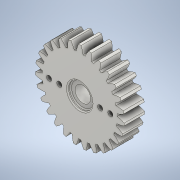
# Autodesk Inventor part: шестерня_1
Saved by Autodesk Inventor 2022 (Build 260153000, 153)
## iProperties
CustomPartVersion: 1
Created: 2022-12-27
Part Number: шестерня_1
Material: Steel
Document SubType Name: Modeling
Designer: Pavel
Categories: <?xml version="1.0" encoding="UTF-16"?> <MemberInstance><Categories><FamilyTemplate><FamilyTemplateParameter ValueType="xs:double" Id="1" ObjectReferenceKey="da_z" ObjectType="kUserParameterObject"/><FamilyTemplateParameter ValueType="xs:double" Id="2" ObjectReferenceKey="da_b" ObjectType="kUserParameterObject"/><FamilyTemplateParameter ValueType="xs:double" Id="3" ObjectReferenceKey="da_beta" ObjectType="kUserParameterObject"/><FamilyTemplateParameter ValueType="xs:double" Id="4" ObjectReferenceKey="da_da" ObjectType="kUserParameterObject"/><FamilyTemplateParameter ValueType="xs:double" Id="5" ObjectReferenceKey="da_aw" ObjectType="kUserParameterObject"/><FamilyTemplateParameter ValueType="xs:string" Id="6" ObjectReferenceKey="EAIAABAAAACIAQAAAAAAAIAAAAAAAAAA" ObjectType="83910656" SubObjectId="SurfaceGeometry"/></FamilyTemplate><ParamToTemplateMap><ParamToTemplate CategoryParameter="//CategoryParameter[@InternalName='046C89C9-8512-4d59-83FE-43B91F4F132A']" TemplateParameter="1"/><ParamToTemplate CategoryParameter="//CategoryParameter[@InternalName='2552DF32-E462-4b46-AEBF-C6C7768E72AC']" TemplateParameter="2"/><ParamToTemplate CategoryParameter="//CategoryParameter[@InternalName='C9EE641D-15FC-4fae-A226-E94C4372FDD7']" TemplateParameter="3"/><ParamToTemplate><ParamToTemplate CategoryParameter="//CategoryParameter[@InternalName='00B6519A-459B-49c7-AD84-2E56D39A5744']" ConstantValue="0.000000"/></ParamToTemplate><ParamToTemplate><ParamToTemplate CategoryParameter="//CategoryParameter[@InternalName='04B31F0E-C7A6-4894-AA32-9629BEFACF47']" ConstantValue="1.000000"/></ParamToTemplate><ParamToTemplate><ParamToTemplate CategoryParameter="//CategoryParameter[@InternalName='43CBEC2E-7847-49e7-A936-2F7889FCB2D9']" ConstantValue="0.250000"/></ParamToTemplate><ParamToTemplate><ParamToTemplate CategoryParameter="//CategoryParameter[@InternalName='B1EFC894-105D-4ebd-86BF-FA20ED196853']" ConstantValue="0.350000"/></ParamToTemplate><ParamToTemplate><ParamToTemplate CategoryParameter="//CategoryParameter[@InternalName='51175063-3D10-4879-93E8-6246FE8B403D']" ConstantValue="2060000000.000000"/></ParamToTemplate><ParamToTemplate><ParamToTemplate CategoryParameter="//CategoryParameter[@InternalName='A3A52E27-4454-46a9-B0BD-C932399B70AF']" ConstantValue="0.300000"/></ParamToTemplate><ParamToTemplate><ParamToTemplate CategoryParameter="//CategoryParameter[@InternalName='91B76062-C214-41d9-B1B9-14D2AB99603D']" ConstantValue="0.150000"/></ParamToTemplate><ParamToTemplate><ParamToTemplate CategoryParameter="//CategoryParameter[@InternalName='374E806E-8B8A-4dda-A9AA-1039D6500AD2']" ConstantValue="6.666667"/></ParamToTemplate><ParamToTemplate><ParamToTemplate CategoryParameter="//CategoryParameter[@InternalName='2D373A89-B862-43d6-8D0B-0CBF12AB9F6C']" ConstantValue="0.349066"/></ParamToTemplate><ParamToTemplate CategoryParameter="//CategoryParameter[@InternalName='37777632-D6A2-4fac-9D53-DB8ACD95C989']" TemplateParameter="4"/><ParamToTemplate CategoryParameter="//CategoryParameter[@InternalName='FD1017F1-B727-4f7e-9707-0F86F1FF9423']" TemplateParameter="5"/><ParamToTemplate><ParamToTemplate CategoryParameter="//CategoryParameter[@InternalName='9E1B4470-B2D3-4ff1-B813-535BB4CDF51A']" ConstantValue="3520000.000000"/></ParamToTemplate><ParamToTemplate><ParamToTemplate CategoryParameter="//CategoryParameter[@InternalName='F8452263-BFF6-458c-9FB1-07C4B99E95CD']" ConstantValue="11400000.000000"/></ParamToTemplate><ParamToTemplate><ParamToTemplate CategoryParameter="//CategoryParameter[@InternalName='3E3BB259-FD49-497f-8171-6EBC954A3479']" ConstantValue="2.000000"/></ParamToTemplate><ParamToTemplate CategoryParameter="//CategoryParameter[@InternalName='27C3BAF2-7550-4e4b-AE2C-0DB134B7D9B7']" TemplateParameter="6"/></ParamToTemplateMap><Category DisplayName="Gear" InternalName="DC85795E-93AB-48d5-8EEE-5A27447B64BD" Mnemonic="Gear"><CategoryParameter DisplayName="z" InternalName="046C89C9-8512-4d59-83FE-43B91F4F132A" Mnemonic="z"/><CategoryParameter DisplayName="b" InternalName="2552DF32-E462-4b46-AEBF-C6C7768E72AC" Mnemonic="b"/><CategoryParameter DisplayName="||b|" InternalName="C9EE641D-15FC-4fae-A226-E94C4372FDD7" Mnemonic="beta"/><CategoryParameter DisplayName="x" InternalName="00B6519A-459B-49c7-AD84-2E56D39A5744" Mnemonic="x"/><CategoryParameter DisplayName="a*" InternalName="04B31F0E-C7A6-4894-AA32-9629BEFACF47" Mnemonic="a"/><CategoryParameter DisplayName="c*" InternalName="43CBEC2E-7847-49e7-A936-2F7889FCB2D9" Mnemonic="c"/><CategoryParameter DisplayName="r|.f|*" InternalName="B1EFC894-105D-4ebd-86BF-FA20ED196853" Mnemonic="rf"/><CategoryParameter DisplayName="E" InternalName="51175063-3D10-4879-93E8-6246FE8B403D" Mnemonic="E"/><CategoryParameter DisplayName="||m|" InternalName="A3A52E27-4454-46a9-B0BD-C932399B70AF" Mnemonic="mi"/><Category DisplayName="SpurGear" InternalName="26C5A22E-A91E-4dfd-A3B3-23CCAFAE1764" Mnemonic="SpurGear"><CategoryParameter DisplayName="m" InternalName="91B76062-C214-41d9-B1B9-14D2AB99603D" Mnemonic="m"/><CategoryParameter DisplayName="P" InternalName="374E806E-8B8A-4dda-A9AA-1039D6500AD2" Mnemonic="PP"/><CategoryParameter DisplayName="||a|" InternalName="2D373A89-B862-43d6-8D0B-0CBF12AB9F6C" Mnemonic="alpha"/><CategoryParameter DisplayName="d|.a|" InternalName="37777632-D6A2-4fac-9D53-DB8ACD95C989" Mnemonic="da"/><CategoryParameter DisplayName="a|.w|" InternalName="FD1017F1-B727-4f7e-9707-0F86F1FF9423" Mnemonic="aw"/><CategoryParameter DisplayName="||s||.Flim|" InternalName="9E1B4470-B2D3-4ff1-B813-535BB4CDF51A" Mnemonic="sFlim"/><CategoryParameter DisplayName="||s||.Hlim|" InternalName="F8452263-BFF6-458c-9FB1-07C4B99E95CD" Mnemonic="sHlim"/><CategoryParameter DisplayName="тип" InternalName="3E3BB259-FD49-497f-8171-6EBC954A3479" Mnemonic="type"/><CategoryParameter DisplayName="PitchDiameter" InternalName="27C3BAF2-7550-4e4b-AE2C-0DB134B7D9B7" Mnemonic="IDS_PITCHDIAM"/></Category></Category></Categories></MemberInstance>
Density: 1 g/cm^3
Appearance: Steel
Author: Pavel
Autodesk Inventor part; units mm, degrees
ref_plane "YZ Plane" through (0, 0, 0) normal (1, 0, 0) x (0, 1, 0)
ref_plane "XZ Plane" through (0, 0, 0) normal (0, 1, 0) x (-1, 0, 0)
ref_plane "XY Plane" through (0, 0, 0) normal (0, 0, 1) x (1, 0, 0)
sketch "Sketch1" plane through (0, 0, 0) normal (0, 0, 1) x (1, 0, 0)
  circle A0 centre (0, 0) radius 21.7404
  dimension "d0" = 43.4808
  constraints: 1 centre point
  measures "d0" diameter of A0
extrude "Extrusion1" add sketch "Sketch1" along normal blind 6
ref_plane "Work Plane2" through (0, 0, 3) normal (0, 0, 1) x (1, 0, 0)
sketch "Sketch2" plane through (0, 0, 0) normal (0, 0, -1) x (-1, 0, 0)
  circle A0 centre (0, 0) radius 21.7404 projected
  circle A1 centre (0, 0) radius 20.25
  dimension "d3" = 40.5
  constraints: 1 centre point, 1 coincident
  measures "d3" diameter of A1
surface extrude "Средний диаметр" sketch "Sketch2" against normal through all shown no curves A1
ref_plane "Work Plane8" through (0, 0, 0) normal (0.9932384, 0.1160929, 0) x (0, 0, 1)
ref_plane "Work Plane9" through (0, 0, 0) normal (1, 0, 0) x (0, 1, 0)
spur gear teeth "Цилиндрическое зубчатое зацепление" teeth 27 pitch diameter 40.5 tip diameter 43.4808 root diameter 36.75 face width 6 start plane through (0, 0, 0) normal (0, 0, -1) x (-1, 0, 0)
sketch "Эскиз6" plane through (0, 0, 6) normal (0, 0, 1) x (1, 0, 0)
  arc A0 (-5.6268, 20.9996) -> (-5.7798, 17.4423) centre (8.4688, 18.6117) ccw projected
  arc A1 (-5.7798, 17.4423) -> (-6.7842, 17.0768) centre (0, 0) ccw projected
  arc A2 (-6.7842, 17.0768) -> (-9.1879, 19.7035) centre (-18.4509, 8.8138) ccw projected
  arc A3 (-9.1879, 19.7035) -> (-10.318, 19.1359) centre (0, 0) ccw projected
  arc A4 (-10.318, 19.1359) -> (-9.6464, 15.6393) centre (3.9483, 20.0631) ccw projected
  arc A5 (-9.6464, 15.6393) -> (-10.5395, 15.0519) centre (0, 0) ccw projected
  arc A6 (-10.5395, 15.0519) -> (-13.4842, 17.0535) centre (-19.9861, 4.3212) ccw projected
  arc A7 (-13.4842, 17.0535) -> (-14.4529, 16.2406) centre (0, 0) ccw projected
  arc A8 (-14.4529, 16.2406) -> (-12.9931, 12.9931) centre (-0.785, 20.4328) ccw projected
  arc A9 (-12.9931, 12.9931) -> (-13.7266, 12.2156) centre (0, 0) ccw projected
  arc A10 (-13.7266, 12.2156) -> (-17.0535, 13.4842) centre (-20.4439, -0.4044) ccw projected
  arc A11 (-17.0535, 13.4842) -> (-17.8087, 12.4698) centre (0, 0) ccw projected
  arc A12 (-17.8087, 12.4698) -> (-15.6393, 9.6464) centre (-5.4759, 19.7011) ccw projected
  arc A13 (-15.6393, 9.6464) -> (-16.1737, 8.7208) centre (0, 0) ccw projected
  arc A14 (-16.1737, 8.7208) -> (-19.7035, 9.1879) centre (-19.7996, -5.1082) ccw projected
  arc A15 (-19.7035, 9.1879) -> (-20.2044, 8.0267) centre (0, 0) ccw projected
  arc A16 (-20.2044, 8.0267) -> (-17.4423, 5.7798) centre (-9.8717, 17.9072) ccw projected
  arc A17 (-17.4423, 5.7798) -> (-17.7489, 4.7558) centre (0, 0) ccw projected
  arc A18 (-17.7489, 4.7558) -> (-21.2913, 4.3963) centre (-18.0878, -9.5366) ccw projected
  arc A19 (-21.2913, 4.3963) -> (-21.5109, 3.1509) centre (0, 0) ccw projected
  arc A20 (-21.5109, 3.1509) -> (-18.3051, 1.6015) centre (-13.7353, 15.1479) ccw projected
  arc A21 (-18.3051, 1.6015) -> (-18.3672, 0.5344) centre (0, 0) ccw projected
  arc A22 (-18.3672, 0.5344) -> (-21.7312, -0.6323) centre (-15.401, -13.4509) ccw projected
  arc A23 (-21.7312, -0.6323) -> (-21.6577, -1.8948) centre (0, 0) ccw projected
  arc A24 (-21.6577, -1.8948) -> (-18.181, -2.6631) centre (-16.8584, 11.572) ccw projected
  arc A25 (-18.181, -2.6631) -> (-17.9954, -3.7157) centre (0, 0) ccw projected
  arc A26 (-17.9954, -3.7157) -> (-20.9996, -5.6268) centre (-11.8838, -16.6401) ccw projected
  arc A27 (-20.9996, -5.6268) -> (-20.6369, -6.8383) centre (0, 0) ccw projected
  arc A28 (-20.6369, -6.8383) -> (-17.0768, -6.7842) centre (-19.0727, 7.3723) ccw projected
  arc A29 (-17.0768, -6.7842) -> (-16.6534, -7.7656) centre (0, 0) ccw projected
  arc A30 (-16.6534, -7.7656) -> (-19.1359, -10.318) centre (-7.7261, -18.9321) ccw projected
  arc A31 (-19.1359, -10.318) -> (-18.5036, -11.4132) centre (0, 0) ccw projected
  arc A32 (-18.5036, -11.4132) -> (-15.0519, -10.5395) centre (-20.2587, 2.7751) ccw projected
  arc A33 (-15.0519, -10.5395) -> (-14.4136, -11.3968) centre (0, 0) ccw projected
  arc A34 (-14.4136, -11.3968) -> (-16.2406, -14.4529) centre (-3.1518, -20.2036) ccw projected
  arc A35 (-16.2406, -14.4529) -> (-15.3728, -15.3728) centre (0, 0) ccw projected
  arc A36 (-15.3728, -15.3728) -> (-12.2156, -13.7266) centre (-20.3526, -1.9717) ccw projected
  arc A37 (-12.2156, -13.7266) -> (-11.3968, -14.4136) centre (0, 0) ccw projected
  arc A38 (-11.3968, -14.4136) -> (-12.4698, -17.8087) centre (1.5925, -20.3858) ccw projected
  arc A39 (-12.4698, -17.8087) -> (-11.4132, -18.5036) centre (0, 0) ccw projected
  arc A40 (-11.4132, -18.5036) -> (-8.7208, -16.1737) centre (-19.3493, -6.6122) ccw projected
  arc A41 (-8.7208, -16.1737) -> (-7.7656, -16.6534) centre (0, 0) ccw projected
  arc A42 (-7.7656, -16.6534) -> (-8.0267, -20.2044) centre (6.2508, -19.4691) ccw projected
  arc A43 (-8.0267, -20.2044) -> (-6.8383, -20.6369) centre (0, 0) ccw projected
  arc A44 (-6.8383, -20.6369) -> (-4.7558, -17.7489) centre (-17.3029, -10.8962) ccw projected
  arc A45 (-4.7558, -17.7489) -> (-3.7157, -17.9954) centre (0, 0) ccw projected
  arc A46 (-3.7157, -17.9954) -> (-3.1509, -21.5109) centre (10.5722, -17.5027) ccw projected
  arc A47 (-3.1509, -21.5109) -> (-1.8948, -21.6577) centre (0, 0) ccw projected
  arc A48 (-1.8948, -21.6577) -> (-0.5344, -18.3672) centre (-14.3236, -14.5928) ccw projected
  arc A49 (-0.5344, -18.3672) -> (0.5344, -18.3672) centre (0, 0) ccw projected
  arc A50 (0.5344, -18.3672) -> (1.8948, -21.6577) centre (14.3236, -14.5928) ccw projected
  arc A51 (1.8948, -21.6577) -> (3.1509, -21.5109) centre (0, 0) ccw projected
  arc A52 (3.1509, -21.5109) -> (3.7157, -17.9954) centre (-10.5722, -17.5027) ccw projected
  arc A53 (3.7157, -17.9954) -> (4.7558, -17.7489) centre (0, 0) ccw projected
  arc A54 (4.7558, -17.7489) -> (6.8383, -20.6369) centre (17.3029, -10.8962) ccw projected
  arc A55 (6.8383, -20.6369) -> (8.0267, -20.2044) centre (0, 0) ccw projected
  arc A56 (8.0267, -20.2044) -> (7.7656, -16.6534) centre (-6.2508, -19.4691) ccw projected
  arc A57 (7.7656, -16.6534) -> (8.7208, -16.1737) centre (0, 0) ccw projected
  arc A58 (8.7208, -16.1737) -> (11.4132, -18.5036) centre (19.3493, -6.6122) ccw projected
  arc A59 (11.4132, -18.5036) -> (12.4698, -17.8087) centre (0, 0) ccw projected
  arc A60 (12.4698, -17.8087) -> (11.3968, -14.4136) centre (-1.5925, -20.3858) ccw projected
  arc A61 (11.3968, -14.4136) -> (12.2156, -13.7266) centre (0, 0) ccw projected
  arc A62 (12.2156, -13.7266) -> (15.3728, -15.3728) centre (20.3526, -1.9717) ccw projected
  arc A63 (15.3728, -15.3728) -> (16.2406, -14.4529) centre (0, 0) ccw projected
  arc A64 (16.2406, -14.4529) -> (14.4136, -11.3968) centre (3.1518, -20.2036) ccw projected
  arc A65 (14.4136, -11.3968) -> (15.0519, -10.5395) centre (0, 0) ccw projected
  arc A66 (15.0519, -10.5395) -> (18.5036, -11.4132) centre (20.2587, 2.7751) ccw projected
  arc A67 (18.5036, -11.4132) -> (19.1359, -10.318) centre (0, 0) ccw projected
  arc A68 (19.1359, -10.318) -> (16.6534, -7.7656) centre (7.7261, -18.9321) ccw projected
  arc A69 (16.6534, -7.7656) -> (17.0768, -6.7842) centre (0, 0) ccw projected
  arc A70 (17.0768, -6.7842) -> (20.6369, -6.8383) centre (19.0727, 7.3723) ccw projected
  arc A71 (20.6369, -6.8383) -> (20.9996, -5.6268) centre (0, 0) ccw projected
  arc A72 (20.9996, -5.6268) -> (17.9954, -3.7157) centre (11.8838, -16.6401) ccw projected
  arc A73 (17.9954, -3.7157) -> (18.181, -2.6631) centre (0, 0) ccw projected
  arc A74 (18.181, -2.6631) -> (21.6577, -1.8948) centre (16.8584, 11.572) ccw projected
  arc A75 (21.6577, -1.8948) -> (21.7312, -0.6323) centre (0, 0) ccw projected
  arc A76 (21.7312, -0.6323) -> (18.3672, 0.5344) centre (15.401, -13.4509) ccw projected
  arc A77 (18.3672, 0.5344) -> (18.3051, 1.6015) centre (0, 0) ccw projected
  arc A78 (18.3051, 1.6015) -> (21.5109, 3.1509) centre (13.7353, 15.1479) ccw projected
  arc A79 (21.5109, 3.1509) -> (21.2913, 4.3963) centre (0, 0) ccw projected
  arc A80 (21.2913, 4.3963) -> (17.7489, 4.7558) centre (18.0878, -9.5366) ccw projected
  arc A81 (17.7489, 4.7558) -> (17.4423, 5.7798) centre (0, 0) ccw projected
  arc A82 (17.4423, 5.7798) -> (20.2044, 8.0267) centre (9.8717, 17.9072) ccw projected
  arc A83 (20.2044, 8.0267) -> (19.7035, 9.1879) centre (0, 0) ccw projected
  arc A84 (19.7035, 9.1879) -> (16.1737, 8.7208) centre (19.7996, -5.1082) ccw projected
  arc A85 (16.1737, 8.7208) -> (15.6393, 9.6464) centre (0, 0) ccw projected
  arc A86 (15.6393, 9.6464) -> (17.8087, 12.4698) centre (5.4759, 19.7011) ccw projected
  arc A87 (17.8087, 12.4698) -> (17.0535, 13.4842) centre (0, 0) ccw projected
  arc A88 (17.0535, 13.4842) -> (13.7266, 12.2156) centre (20.4439, -0.4044) ccw projected
  arc A89 (13.7266, 12.2156) -> (12.9931, 12.9931) centre (0, 0) ccw projected
  arc A90 (12.9931, 12.9931) -> (14.4529, 16.2406) centre (0.785, 20.4328) ccw projected
  arc A91 (14.4529, 16.2406) -> (13.4842, 17.0535) centre (0, 0) ccw projected
  arc A92 (13.4842, 17.0535) -> (10.5395, 15.0519) centre (19.9861, 4.3212) ccw projected
  arc A93 (10.5395, 15.0519) -> (9.6464, 15.6393) centre (0, 0) ccw projected
  arc A94 (9.6464, 15.6393) -> (10.318, 19.1359) centre (-3.9483, 20.0631) ccw projected
  arc A95 (10.318, 19.1359) -> (9.1879, 19.7035) centre (0, 0) ccw projected
  arc A96 (9.1879, 19.7035) -> (6.7842, 17.0768) centre (18.4509, 8.8138) ccw projected
  arc A97 (6.7842, 17.0768) -> (5.7798, 17.4423) centre (0, 0) ccw projected
  arc A98 (5.7798, 17.4423) -> (5.6268, 20.9996) centre (-8.4688, 18.6117) ccw projected
  arc A99 (5.6268, 20.9996) -> (4.3963, 21.2913) centre (0, 0) ccw projected
  arc A100 (4.3963, 21.2913) -> (2.6631, 18.181) centre (15.9209, 12.8313) ccw projected
  arc A101 (2.6631, 18.181) -> (1.6015, 18.3051) centre (0, 0) ccw projected
  arc A102 (1.6015, 18.3051) -> (0.6323, 21.7312) centre (-12.5327, 16.157) ccw projected
  arc A103 (0.6323, 21.7312) -> (-0.6323, 21.7312) centre (0, 0) ccw projected
  arc A104 (-0.6323, 21.7312) -> (-1.6015, 18.3051) centre (12.5327, 16.157) ccw projected
  arc A105 (-1.6015, 18.3051) -> (-2.6631, 18.181) centre (0, 0) ccw projected
  arc A106 (-2.6631, 18.181) -> (-4.3963, 21.2913) centre (-15.9209, 12.8313) ccw projected
  arc A107 (-4.3963, 21.2913) -> (-5.6268, 20.9996) centre (0, 0) ccw projected
extrude "Выдавливание5" add sketch "Эскиз6" along normal blind 4
sketch "Эскиз4" plane through (0, 0, 6) normal (0, 0, 1) x (1, 0, 0)
  circle A0 centre (0, 0) radius 3.8
  line L0 (0, 0) -> (10, 0) construction
  circle A1 centre (10, 0) radius 1.25
  line L1 (10, 0) -> (15, 0) construction
  circle A2 centre (15, 0) radius 1.25
  circle A3 centre (-10, 0) radius 1.25
  circle A4 centre (-15, 0) radius 1.25
  dimension "d52" = 7.6
  dimension "d53" = 10
  dimension "d54" = 2.5
  dimension "d55" = 5
  dimension "d58" = 360
  constraints: 5 centre point, 4 end point, 3 coincident, 2 horizontal, 1 equal radius, 9 other
  measures "d52" diameter of A0
  measures "d53" distance of L0.start L0.end
  measures "d54" diameter of A1
  measures "d55" distance of L1.start L1.end
extrude "Выдавливание3" cut sketch "Эскиз4" along normal mid plane 100
sketch "Эскиз5" plane through (0, 0, 0) normal (0, 0, -1) x (-1, 0, 0)
  circle A0 centre (-15, 0) radius 1.25 projected
  line L0 (-12.4, 1.5011) -> (-12.4, -1.5011)
  line L1 (-12.4, -1.5011) -> (-15, -3.0022)
  line L2 (-15, -3.0022) -> (-17.6, -1.5011)
  line L3 (-17.6, -1.5011) -> (-17.6, 1.5011)
  line L4 (-17.6, 1.5011) -> (-15, 3.0022)
  line L5 (-15, 3.0022) -> (-12.4, 1.5011)
  circle A1 centre (-10, 0) radius 1.25 projected
  line L6 (-7.4, -1.5011) -> (-10, -3.0022)
  line L7 (-10, -3.0022) -> (-12.6, -1.5011)
  line L8 (-12.6, -1.5011) -> (-12.6, 1.5011)
  line L9 (-12.6, 1.5011) -> (-10, 3.0022)
  line L10 (-10, 3.0022) -> (-7.4, 1.5011)
  line L11 (-7.4, 1.5011) -> (-7.4, -1.5011)
  line L12 (7.4, -1.5011) -> (7.4, 1.5011)
  line L13 (7.4, 1.5011) -> (10, 3.0022)
  line L14 (10, -3.0022) -> (7.4, -1.5011)
  line L15 (10, 3.0022) -> (12.6, 1.5011)
  line L16 (12.6, -1.5011) -> (10, -3.0022)
  line L17 (12.4, -1.5011) -> (12.4, 1.5011)
  line L18 (12.6, 1.5011) -> (12.6, -1.5011)
  line L19 (12.4, 1.5011) -> (15, 3.0022)
  line L20 (15, -3.0022) -> (12.4, -1.5011)
  line L21 (15, 3.0022) -> (17.6, 1.5011)
  line L22 (17.6, 1.5011) -> (17.6, -1.5011)
  line L23 (17.6, -1.5011) -> (15, -3.0022)
  point P0 (0, 0)
  point P1 (-7.4, 0)
  point P2 (7.4, 0)
  point P3 (10, 0)
  point P4 (15, 0)
  point P5 (12.5, 1.5588)
  point P6 (12.5, -1.5588)
  point P7 (-12.5, -1.5588)
  point P8 (-12.5, 1.5588)
  dimension "d62" = 5.2
  dimension "d69" = 5.2
  dimension "d72" = 360
  constraints: 48 end point, 2 coincident, 1 midpoint, 1 vertical, 1 vertical alignment, 81 other
  measures "d62" distance between parallel lines of L0 L3
  measures "d69" distance between parallel lines of L11 L8
extrude "Выдавливание4" cut sketch "Эскиз5" against normal blind 1.5 contours A0 | L5 L9 L10 L11 L6 L7 L1 L0 | L0 L1 L7 L8 L9 L5 | L9 L8 L7 L1 L2 L3 L4 L5 | L12 L13 L15 L19 L17 L20 L16 L14 | L20 L17 L19 L15 L18 L16 | L16 L18 L15 L19 L21 L22 L23 L20
sketch "Эскиз7" plane through (0, 0, 10) normal (0, 0, 1) x (1, 0, 0)
  circle A0 centre (0, 0) radius 3.8 projected
  circle A1 centre (0, 0) radius 6
  dimension "d76" = 12
  constraints: 1 centre point, 1 coincident
  measures "d76" diameter of A1
extrude "Выдавливание6" cut sketch "Эскиз7" against normal blind 1.5
fillet "Сопряжение1" radius 0.5 2 edges at (-6, 0, 10) (-6, 0, 8.5)
equation "\"d0\" = da_da"
equation "\"d1\" = da_b"
equation "\"d3\" = da_d"
equation "\"d16\" = da_aw"
equation "\"d43\" = da_aw"
equation "\"d46\" = da_aw"
equation "\"da_da\" = 43.480844"
equation "\"da_b\" = 6"
equation "\"da_d\" = 40.5"
equation "\"da_aw\" = 40.825"
body "Solid1"
body "Srf1"
